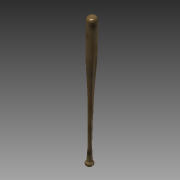
# Autodesk Inventor part: Baseball Bat
Saved by Autodesk Inventor 2015 (Build 190159000, 159)
## iProperties
Created: 2016-04-09
Part Number: Baseball Bat
Material: Generic
Document SubType Name: Modeling
Designer: tquinn
Density: 1 g/cm^3
Appearance: Default
Author: tquinn
Autodesk Inventor part; units mm, degrees
ref_plane "YZ Plane" through (0, 0, 0) normal (1, 0, 0) x (0, 1, 0)
ref_plane "XZ Plane" through (0, 0, 0) normal (0, 1, 0) x (-1, 0, 0)
ref_plane "XY Plane" through (0, 0, 0) normal (0, 0, 1) x (1, 0, 0)
sketch "Sketch1" plane through (0, 0, 0) normal (0, 0, 1) x (1, 0, 0)
  line L0 (-30.3345, 130.8414) -> (42.1735, 130.8414) construction
  line L1 (42.1735, 130.8414) -> (42.1735, -3.4075) construction
  line L2 (42.1735, -3.4075) -> (-30.3345, -3.4075) construction
  line L3 (-30.3345, -3.4075) -> (-30.3345, 130.8414) construction
  line L4 (6.9014, 127.4271) -> (4.2732, 0.4271)
  line L5 (6.9014, 127.4271) -> (8.1492, 127.4271)
  line L6 (11.2293, 124.8252) -> (10.3505, 95.1017)
  arc A0 (11.2293, 124.8252) -> (8.1492, 127.4271) centre (8.1492, 124.3031) ccw
  line L7 (7.61, 2.7168) -> (7.5887, 1.6884)
  line L8 (4.2732, 0.4271) -> (7.3741, 0.3629)
  line L9 (7.5887, 1.6884) -> (7.5612, 0.3591)
  line L10 (7.5612, 0.3591) -> (7.3741, 0.3629)
  spline S0 degree 4 poles (6.587, 3.8378) (6.2712, 5.8409) (6.6041, 7.9563) (5.9817, 15.2538) (6.1665, 19.925) (6.6199, 28.5532) (6.5506, 36.3142) (7.2472, 44.6161) (7.335, 55.224) (8.6917, 71.9737) (9.6285, 83.6593) (10.4095, 93.0312) (10.3505, 95.1017) knots 0 0 0 0 0 0.147536 0.218232 0.296166 0.378355 0.469747 0.568392 0.672557 0.779311 1 1 1 1 1
  line L11 (6.9014, 127.4271) -> (4.2732, 0.4271)
  line L12 (4.2732, 0.4271) -> (7.5612, 0.3591)
  line L13 (7.5612, 0.3591) -> (7.61, 2.7168)
  line L14 (6.587, 3.8378) -> (7.61, 2.7168)
  line L15 (10.3505, 95.1017) -> (10.3505, 95.1017)
  point P0 (10.1652, 126.6895)
  point P1 (6.4077, 6.4455)
  point P2 (6.3449, 10.2492)
  point P3 (6.1367, 15.513)
  point P4 (6.1805, 19.8067)
  point P5 (6.4933, 27.514)
  point P6 (6.6812, 35.8156)
  point P7 (7.0731, 43.8868)
  point P8 (7.4743, 54.4812)
  point P9 (8.3882, 68.2194)
  point P10 (9.4255, 81.0774)
  point P11 (10.1904, 91.1338)
  dimension "d3" = 134.249
  dimension "d20" = 127
  constraints: 24 end point, 3 perpendicular, 3 point on circle, 2 collinear, 1 centre point, 1 horizontal, 1 point on line, 1 tangent, 1 vertical, 20 other
  measures "d3" distance of L2.end L0.start
  measures "d20" vertical distance of L4.start L4.end
revolve "Revolution2" add sketch "Sketch1" angle 360 about axis through (6.9014, 127.4271, 0) along (-0.02069, -0.9997859, 0)
fillet "Fillet1" radius 0.7937 1 edges at (0.9852, 0.4951, 0)
equation "\"d3\" = 1.05708 * d20"
body "Solid2"
